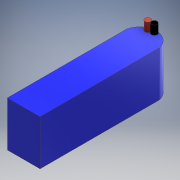
# Autodesk Inventor part: turnigy_sa
Saved by Autodesk Inventor 2018 (Build 220112000, 112)
## iProperties
Created: 2018-03-07
Part Number: turnigy_sa
Material: 一般
Document SubType Name: Modeling
Designer: shun
Density: 1 g/cm^3
Appearance: 既定
Author: shun
Autodesk Inventor part; units mm, degrees
ref_plane "YZ Plane" through (0, 0, 0) normal (1, 0, 0) x (0, 1, 0)
ref_plane "XZ Plane" through (0, 0, 0) normal (0, 1, 0) x (-1, 0, 0)
ref_plane "XY Plane" through (0, 0, 0) normal (0, 0, 1) x (1, 0, 0)
sketch "スケッチ1" plane through (0, 0, 0) normal (0, 0, 1) x (1, 0, 0)
  line L0 (0, 0) -> (37, 0)
  line L1 (37, 0) -> (37, 135)
  line L2 (0, 135) -> (0, 0)
  arc A0 (37, 135) -> (0, 135) centre (18.5, 131.0917) ccw
  point P0 (18.5, 150)
  dimension "d0" = 37
  dimension "d1" = 135
  constraints: 6 end point, 3 point on circle, 1 centre point, 1 horizontal, 1 parallel, 1 perpendicular
  measures "d0" distance of L2.start L1.end
  measures "d1" distance of L1.end L0.end
extrude "押し出し1" add sketch "スケッチ1" along normal blind 51
sketch "スケッチ2" plane through (0, 0, 51) normal (0, 0, 1) x (1, 0, 0)
  circle A0 centre (13.1184, 145.7961) radius 3.25
  circle A1 centre (19.5531, 146.7145) radius 3.25
  arc A2 (37, 135) -> (0, 135) centre (18.5, 131.0917) ccw projected
  point P0 (0, 0)
  dimension "d5" = 6.5
  dimension "d6" = 6.5
  constraints: 3 tangent, 2 centre point
  measures "d5" diameter of A0
  measures "d6" diameter of A1
extrude "押し出し2" add sketch "スケッチ2" along normal blind 10 contours A0 | A1
